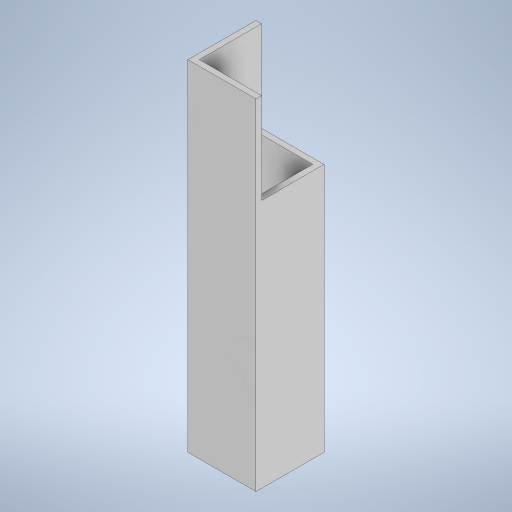
# Autodesk Inventor part: testRoboRescue_Chassis_Frame_heightBar
Saved by Autodesk Inventor 2023 (Build 270158000, 158)
## iProperties
Created: 2022-03-14
Part Number: testRoboRescue_Chassis_Frame_heightBar
Material: Aluminum 6061
Document SubType Name: Modeling
Designer: Nebil Oumer
Density: 2.7 g/cm^3
Appearance: Aluminum - Polished
Mass: 199.103 g
Surface Area: 476.612 cm^2
Volume: 73.7418 cm^3
Author: Nebil Oumer
Autodesk Inventor part; units mm, degrees
ref_plane "YZ Plane" through (0, 0, 0) normal (1, 0, 0) x (0, 1, 0)
ref_plane "XZ Plane" through (0, 0, 0) normal (0, 1, 0) x (-1, 0, 0)
ref_plane "XY Plane" through (0, 0, 0) normal (0, 0, 1) x (1, 0, 0)
sketch "Sketch2" plane through (0, 0, 0) normal (0, 0, 1) x (1, 0, 0)
  line L0 (0, 0) -> (38.1, 0)
  line L1 (38.1, 0) -> (38.1, 38.1)
  line L2 (38.1, 38.1) -> (0, 38.1)
  line L3 (0, 38.1) -> (0, 0)
  line L4 (3.175, 34.925) -> (34.925, 34.925)
  line L5 (34.925, 34.925) -> (34.925, 3.175)
  line L6 (34.925, 3.175) -> (3.175, 3.175)
  line L7 (3.175, 3.175) -> (3.175, 34.925)
  dimension "d0" = 38.1
  dimension "d1" = 38.1
  dimension "d2" = 3.175
  constraints: 16 end point, 4 parallel, 2 perpendicular, 1 horizontal, 3 other
  measures "d0" distance of L2.end L1.end
  measures "d1" distance of L0.end L1.end
  measures "d2" distance between parallel lines of L2 L4
extrude "Extrusion1" add sketch "Sketch2" along normal blind 139.7
sketch "Sketch3" plane through (0, 0, 139.7) normal (0, 0, 1) x (1, 0, 0)
  line L0 (38.1, 0) -> (38.1, 38.1) projected
  line L1 (38.1, 38.1) -> (0, 38.1) projected
  line L2 (0, 38.1) -> (0, 0) projected
  line L3 (0, 0) -> (38.1, 0) projected
  line L4 (3.175, 34.925) -> (34.925, 34.925) projected
  line L5 (34.925, 34.925) -> (34.925, 3.175) projected
  line L6 (34.925, 3.175) -> (3.175, 3.175) projected
  line L7 (3.175, 3.175) -> (3.175, 34.925) projected
  line L8 (3.175, 34.925) -> (0, 34.925)
  line L9 (34.925, 3.175) -> (34.925, 0)
  constraints: 4 end point, 2 perpendicular, 2 point on line
extrude "Extrusion2" add sketch "Sketch3" along normal blind 50.8 contours L3 L9 L5 L4 L8 L2 L1 L0
equation "\"d0\" = d1"
body "Solid1"
